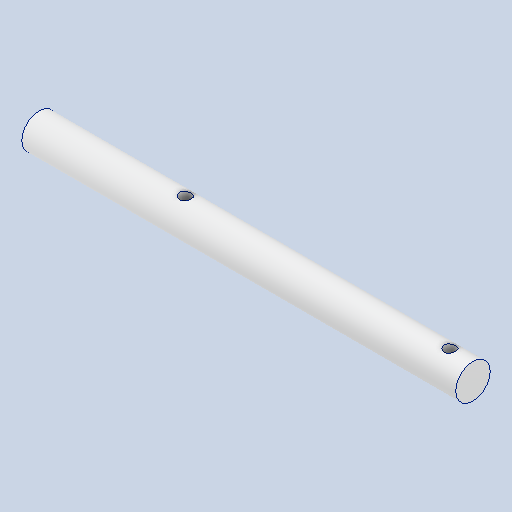
# Autodesk Inventor part: belt_liner_v2_shaft_2
Saved by Autodesk Inventor 2025.2 (Build 292293000, 293)
## iProperties
Created: 2025-01-28
Part Number: belt_liner_v2_shaft_2
Material: アルミニウム 6061
Document SubType Name: Modeling
Designer: haruy
Density: 2.7 g/cm^3
Appearance: アルミニウム - フラット
Author: haruy
Autodesk Inventor part; units mm, degrees
ref_plane "YZ Plane" through (0, 0, 0) normal (1, 0, 0) x (0, 1, 0)
ref_plane "XY Plane" through (0, 0, 0) normal (0, 0, 1) x (1, 0, 0)
sketch "スケッチ1" plane through (0, 0, 0) normal (1, 0, 0) x (0, 1, 0)
  circle A0 centre (0, 0) radius 3
  dimension "d0" = 6
  constraints: 1 centre point, 1 coincident
  measures "d0" diameter of A0
extrude "押し出し1" add sketch "スケッチ1" along normal blind 75.5
ref_plane "作業平面1" through (0, -3, 0) normal (0, 1, 0) x (-1, 0, 0)
sketch "スケッチ2" plane through (0, -3, 0) normal (0, 1, 0) x (-1, 0, 0)
  line L0 (0, 3) -> (0, -3) projected
  point P0 (0, 0)
  point P1 (-25.5, 0)
  point P2 (-71.5, 0)
  dimension "d3" = 25.5
  dimension "d4" = 46
  measures "d3" distance from line of point (-25.5, 0) L0
  measures "d4" distance of point (-25.5, 0) point (-71.5, 0)
hole "穴1" at (25.5, -3, 0) at (71.5, -3, 0) direction (0, 1, 0) diameter 2 end through all
